Autodesk Inventor part; units mm, degrees
(part 4 of 4)
  line L444 (34, -62) -> (25.5, -62) projected
  line L445 (25.5, -62) -> (25.5, -60.5) projected
  line L446 (25.5, -60.5) -> (34, -60.5) projected
  line L447 (34, -60.5) -> (34, -62) projected
  line L448 (49, -32) -> (40.5, -32) projected
  line L449 (40.5, -32) -> (40.5, -30.5) projected
  line L450 (40.5, -30.5) -> (49, -30.5) projected
  line L451 (49, -30.5) -> (49, -32) projected
  line L452 (49, -62) -> (40.5, -62) projected
  line L453 (40.5, -62) -> (40.5, -60.5) projected
  line L454 (40.5, -60.5) -> (49, -60.5) projected
  line L455 (49, -60.5) -> (49, -62) projected
  line L456 (34, 60.5) -> (25.5, 60.5) projected
  line L457 (25.5, 60.5) -> (25.5, 62) projected
  line L458 (25.5, 62) -> (34, 62) projected
  line L459 (34, 62) -> (34, 60.5) projected
  line L460 (49, 58) -> (40.5, 58) projected
  line L461 (40.5, 58) -> (40.5, 59.5) projected
  line L462 (40.5, 59.5) -> (49, 59.5) projected
  line L463 (49, 59.5) -> (49, 58) projected
  line L464 (49, 45.5) -> (40.5, 45.5) projected
  line L465 (40.5, 45.5) -> (40.5, 47) projected
  line L466 (40.5, 47) -> (49, 47) projected
  line L467 (49, 47) -> (49, 45.5) projected
  line L468 (34, 30.5) -> (25.5, 30.5) projected
  line L469 (25.5, 30.5) -> (25.5, 32) projected
  line L470 (25.5, 32) -> (34, 32) projected
  line L471 (34, 32) -> (34, 30.5) projected
  line L472 (49, 43) -> (40.5, 43) projected
  line L473 (40.5, 43) -> (40.5, 44.5) projected
  line L474 (40.5, 44.5) -> (49, 44.5) projected
  line L475 (49, 44.5) -> (49, 43) projected
  line L476 (49, -2) -> (40.5, -2) projected
  line L477 (40.5, -2) -> (40.5, -0.5) projected
  line L478 (40.5, -0.5) -> (49, -0.5) projected
  line L479 (49, -0.5) -> (49, -2) projected
  line L480 (19, 103) -> (10.5, 103) projected
  line L481 (10.5, 103) -> (10.5, 104.5) projected
  line L482 (10.5, 104.5) -> (19, 104.5) projected
  line L483 (19, 104.5) -> (19, 103) projected
  line L484 (34, 103) -> (25.5, 103) projected
  line L485 (25.5, 103) -> (25.5, 104.5) projected
  line L486 (25.5, 104.5) -> (34, 104.5) projected
  line L487 (34, 104.5) -> (34, 103) projected
  line L488 (49, 103) -> (40.5, 103) projected
  line L489 (40.5, 103) -> (40.5, 104.5) projected
  line L490 (40.5, 104.5) -> (49, 104.5) projected
  line L491 (49, 104.5) -> (49, 103) projected
  line L492 (4, 103) -> (-4.5, 103) projected
  line L493 (-4.5, 103) -> (-4.5, 104.5) projected
  line L494 (-4.5, 104.5) -> (4, 104.5) projected
  line L495 (4, 104.5) -> (4, 103) projected
  line L496 (-11, 103) -> (-19.5, 103) projected
  line L497 (-19.5, 103) -> (-19.5, 104.5) projected
  line L498 (-19.5, 104.5) -> (-11, 104.5) projected
  line L499 (-11, 104.5) -> (-11, 103) projected
  line L500 (-26, 103) -> (-34.5, 103) projected
  line L501 (-34.5, 103) -> (-34.5, 104.5) projected
  line L502 (-34.5, 104.5) -> (-26, 104.5) projected
  line L503 (-26, 104.5) -> (-26, 103) projected
  line L504 (-41, 105.5) -> (-49.5, 105.5) projected
  line L505 (-49.5, 105.5) -> (-49.5, 107) projected
  line L506 (-49.5, 107) -> (-41, 107) projected
  line L507 (-41, 107) -> (-41, 105.5) projected
  line L508 (19, -84.5) -> (10.5, -84.5) projected
  line L509 (10.5, -84.5) -> (10.5, -83) projected
  line L510 (10.5, -83) -> (19, -83) projected
  line L511 (19, -83) -> (19, -84.5) projected
  line L512 (19, -39.5) -> (10.5, -39.5) projected
  line L513 (10.5, -39.5) -> (10.5, -38) projected
  line L514 (10.5, -38) -> (19, -38) projected
  line L515 (19, -38) -> (19, -39.5) projected
  line L516 (19, 20.5) -> (10.5, 20.5) projected
  line L517 (10.5, 20.5) -> (10.5, 22) projected
  line L518 (10.5, 22) -> (19, 22) projected
  line L519 (19, 22) -> (19, 20.5) projected
  line L520 (19, 65.5) -> (10.5, 65.5) projected
  line L521 (10.5, 65.5) -> (10.5, 67) projected
  line L522 (10.5, 67) -> (19, 67) projected
  line L523 (19, 67) -> (19, 65.5) projected
  line L524 (19, 43) -> (10.5, 43) projected
  line L525 (10.5, 43) -> (10.5, 44.5) projected
  line L526 (10.5, 44.5) -> (19, 44.5) projected
  line L527 (19, 44.5) -> (19, 43) projected
  line L528 (19, 5.5) -> (10.5, 5.5) projected
  line L529 (10.5, 5.5) -> (10.5, 7) projected
  line L530 (10.5, 7) -> (19, 7) projected
  line L531 (19, 7) -> (19, 5.5) projected
  line L532 (19, -62) -> (10.5, -62) projected
  line L533 (10.5, -62) -> (10.5, -60.5) projected
  line L534 (10.5, -60.5) -> (19, -60.5) projected
  line L535 (19, -60.5) -> (19, -62) projected
  line L536 (19, -99.5) -> (10.5, -99.5) projected
  line L537 (10.5, -99.5) -> (10.5, -98) projected
  line L538 (10.5, -98) -> (19, -98) projected
  line L539 (19, -98) -> (19, -99.5) projected
  line L540 (-26, 118) -> (-34.5, 118) projected
  line L541 (-34.5, 118) -> (-34.5, 119.5) projected
  line L542 (-34.5, 119.5) -> (-26, 119.5) projected
  line L543 (-26, 119.5) -> (-26, 118) projected
  line L544 (-11, 118) -> (-19.5, 118) projected
  line L545 (-19.5, 118) -> (-19.5, 119.5) projected
  line L546 (-19.5, 119.5) -> (-11, 119.5) projected
  line L547 (-11, 119.5) -> (-11, 118) projected
  line L548 (4, 118) -> (-4.5, 118) projected
  line L549 (-4.5, 118) -> (-4.5, 119.5) projected
  line L550 (-4.5, 119.5) -> (4, 119.5) projected
  line L551 (4, 119.5) -> (4, 118) projected
  line L552 (-41, 90.5) -> (-49.5, 90.5) projected
  line L553 (-49.5, 90.5) -> (-49.5, 92) projected
  line L554 (-49.5, 92) -> (-41, 92) projected
  line L555 (-41, 92) -> (-41, 90.5) projected
  line L556 (49, 118) -> (40.5, 118) projected
  line L557 (40.5, 118) -> (40.5, 119.5) projected
  line L558 (40.5, 119.5) -> (49, 119.5) projected
  line L559 (49, 119.5) -> (49, 118) projected
  line L560 (34, 118) -> (25.5, 118) projected
  line L561 (25.5, 118) -> (25.5, 119.5) projected
  line L562 (25.5, 119.5) -> (34, 119.5) projected
  line L563 (34, 119.5) -> (34, 118) projected
  line L564 (19, 118) -> (10.5, 118) projected
  line L565 (10.5, 118) -> (10.5, 119.5) projected
  line L566 (10.5, 119.5) -> (19, 119.5) projected
  line L567 (19, 119.5) -> (19, 118) projected
  line L568 (49, 28) -> (40.5, 28) projected
  line L569 (40.5, 28) -> (40.5, 29.5) projected
  line L570 (40.5, 29.5) -> (49, 29.5) projected
  line L571 (49, 29.5) -> (49, 28) projected
  line L572 (34, 15.5) -> (25.5, 15.5) projected
  line L573 (25.5, 15.5) -> (25.5, 17) projected
  line L574 (25.5, 17) -> (34, 17) projected
  line L575 (34, 17) -> (34, 15.5) projected
  line L576 (34, 45.5) -> (25.5, 45.5) projected
  line L577 (25.5, 45.5) -> (25.5, 47) projected
  line L578 (25.5, 47) -> (34, 47) projected
  line L579 (34, 47) -> (34, 45.5) projected
  line L580 (49, 0.5) -> (40.5, 0.5) projected
  line L581 (40.5, 0.5) -> (40.5, 2) projected
  line L582 (40.5, 2) -> (49, 2) projected
  line L583 (49, 2) -> (49, 0.5) projected
  line L584 (49, 73) -> (40.5, 73) projected
  line L585 (40.5, 73) -> (40.5, 74.5) projected
  line L586 (40.5, 74.5) -> (49, 74.5) projected
  line L587 (49, 74.5) -> (49, 73) projected
  line L588 (34, 75.5) -> (25.5, 75.5) projected
  line L589 (25.5, 75.5) -> (25.5, 77) projected
  line L590 (25.5, 77) -> (34, 77) projected
  line L591 (34, 77) -> (34, 75.5) projected
  line L592 (49, -47) -> (40.5, -47) projected
  line L593 (40.5, -47) -> (40.5, -45.5) projected
  line L594 (40.5, -45.5) -> (49, -45.5) projected
  line L595 (49, -45.5) -> (49, -47) projected
  line L596 (49, -17) -> (40.5, -17) projected
  line L597 (40.5, -17) -> (40.5, -15.5) projected
  line L598 (40.5, -15.5) -> (49, -15.5) projected
  line L599 (49, -15.5) -> (49, -17) projected
  line L600 (34, -47) -> (25.5, -47) projected
  line L601 (25.5, -47) -> (25.5, -45.5) projected
  line L602 (25.5, -45.5) -> (34, -45.5) projected
  line L603 (34, -45.5) -> (34, -47) projected
  line L604 (34, -14.5) -> (25.5, -14.5) projected
  line L605 (25.5, -14.5) -> (25.5, -13) projected
  line L606 (25.5, -13) -> (34, -13) projected
  line L607 (34, -13) -> (34, -14.5) projected
  line L608 (49, -104.5) -> (40.5, -104.5) projected
  line L609 (40.5, -104.5) -> (40.5, -103) projected
  line L610 (40.5, -103) -> (49, -103) projected
  line L611 (49, -103) -> (49, -104.5) projected
  line L612 (34, -119.5) -> (25.5, -119.5) projected
  line L613 (25.5, -119.5) -> (25.5, -118) projected
  line L614 (25.5, -118) -> (34, -118) projected
  line L615 (34, -118) -> (34, -119.5) projected
  line L616 (34, -74.5) -> (25.5, -74.5) projected
  line L617 (25.5, -74.5) -> (25.5, -73) projected
  line L618 (25.5, -73) -> (34, -73) projected
  line L619 (34, -73) -> (34, -74.5) projected
  line L620 (34, 88) -> (25.5, 88) projected
  line L621 (25.5, 88) -> (25.5, 89.5) projected
  line L622 (25.5, 89.5) -> (34, 89.5) projected
  line L623 (34, 89.5) -> (34, 88) projected
  line L624 (-11, -17) -> (-19.5, -17) projected
  line L625 (-19.5, -17) -> (-19.5, -15.5) projected
  line L626 (-19.5, -15.5) -> (-11, -15.5) projected
  line L627 (-11, -15.5) -> (-11, -17) projected
  line L628 (-11, -59.5) -> (-19.5, -59.5) projected
  line L629 (-19.5, -59.5) -> (-19.5, -58) projected
  line L630 (-19.5, -58) -> (-11, -58) projected
  line L631 (-11, -58) -> (-11, -59.5) projected
  line L632 (4, -62) -> (-4.5, -62) projected
  line L633 (-4.5, -62) -> (-4.5, -60.5) projected
  line L634 (-4.5, -60.5) -> (4, -60.5) projected
  line L635 (4, -60.5) -> (4, -62) projected
  line L636 (-11, -44.5) -> (-19.5, -44.5) projected
  line L637 (-19.5, -44.5) -> (-19.5, -43) projected
  line L638 (-19.5, -43) -> (-11, -43) projected
  line L639 (-11, -43) -> (-11, -44.5) projected
  line L640 (-11, -77) -> (-19.5, -77) projected
  line L641 (-19.5, -77) -> (-19.5, -75.5) projected
  line L642 (-19.5, -75.5) -> (-11, -75.5) projected
  line L643 (-11, -75.5) -> (-11, -77) projected
  line L644 (-11, -107) -> (-19.5, -107) projected
  line L645 (-19.5, -107) -> (-19.5, -105.5) projected
  line L646 (-19.5, -105.5) -> (-11, -105.5) projected
  line L647 (-11, -105.5) -> (-11, -107) projected
  line L648 (4, -89.5) -> (-4.5, -89.5) projected
  line L649 (-4.5, -89.5) -> (-4.5, -88) projected
  line L650 (-4.5, -88) -> (4, -88) projected
  line L651 (4, -88) -> (4, -89.5) projected
  line L652 (4, -104.5) -> (-4.5, -104.5) projected
  line L653 (-4.5, -104.5) -> (-4.5, -103) projected
  line L654 (-4.5, -103) -> (4, -103) projected
  line L655 (4, -103) -> (4, -104.5) projected
  line L656 (19, -119.5) -> (10.5, -119.5) projected
  line L657 (10.5, -119.5) -> (10.5, -118) projected
  line L658 (10.5, -118) -> (19, -118) projected
  line L659 (19, -118) -> (19, -119.5) projected
  line L660 (19, 88) -> (10.5, 88) projected
  line L661 (10.5, 88) -> (10.5, 89.5) projected
  line L662 (10.5, 89.5) -> (19, 89.5) projected
  line L663 (19, 89.5) -> (19, 88) projected
  line L664 (4, -77) -> (-4.5, -77) projected
  line L665 (-4.5, -77) -> (-4.5, -75.5) projected
  line L666 (-4.5, -75.5) -> (4, -75.5) projected
  line L667 (4, -75.5) -> (4, -77) projected
  line L668 (-11, -119.5) -> (-19.5, -119.5) projected
  line L669 (-19.5, -119.5) -> (-19.5, -118) projected
  line L670 (-19.5, -118) -> (-11, -118) projected
  line L671 (-11, -118) -> (-11, -119.5) projected
  line L672 (-11, -89.5) -> (-19.5, -89.5) projected
  line L673 (-19.5, -89.5) -> (-19.5, -88) projected
  line L674 (-19.5, -88) -> (-11, -88) projected
  line L675 (-11, -88) -> (-11, -89.5) projected
  line L676 (4, -59.5) -> (-4.5, -59.5) projected
  line L677 (-4.5, -59.5) -> (-4.5, -58) projected
  line L678 (-4.5, -58) -> (4, -58) projected
  line L679 (4, -58) -> (4, -59.5) projected
  line L680 (4, -29.5) -> (-4.5, -29.5) projected
  line L681 (-4.5, -29.5) -> (-4.5, -28) projected
  line L682 (-4.5, -28) -> (4, -28) projected
  line L683 (4, -28) -> (4, -29.5) projected
  line L684 (-11, -62) -> (-19.5, -62) projected
  line L685 (-19.5, -62) -> (-19.5, -60.5) projected
  line L686 (-19.5, -60.5) -> (-11, -60.5) projected
  line L687 (-11, -60.5) -> (-11, -62) projected
  line L688 (-11, -29.5) -> (-19.5, -29.5) projected
  line L689 (-19.5, -29.5) -> (-19.5, -28) projected
  line L690 (-19.5, -28) -> (-11, -28) projected
  line L691 (-11, -28) -> (-11, -29.5) projected
  line L692 (-11, -2) -> (-19.5, -2) projected
  line L693 (-19.5, -2) -> (-19.5, -0.5) projected
  line L694 (-19.5, -0.5) -> (-11, -0.5) projected
  line L695 (-11, -0.5) -> (-11, -2) projected
  line L696 (34, -104.5) -> (25.5, -104.5) projected
  line L697 (25.5, -104.5) -> (25.5, -103) projected
  line L698 (25.5, -103) -> (34, -103) projected
  line L699 (34, -103) -> (34, -104.5) projected
  line L700 (34, -92) -> (25.5, -92) projected
  line L701 (25.5, -92) -> (25.5, -90.5) projected
  line L702 (25.5, -90.5) -> (34, -90.5) projected
  line L703 (34, -90.5) -> (34, -92) projected
  line L704 (49, -89.5) -> (40.5, -89.5) projected
  line L705 (40.5, -89.5) -> (40.5, -88) projected
  line L706 (40.5, -88) -> (49, -88) projected
  line L707 (49, -88) -> (49, -89.5) projected
  line L708 (34, -29.5) -> (25.5, -29.5) projected
  line L709 (25.5, -29.5) -> (25.5, -28) projected
  line L710 (25.5, -28) -> (34, -28) projected
  line L711 (34, -28) -> (34, -29.5) projected
  line L712 (34, -44.5) -> (25.5, -44.5) projected
  line L713 (25.5, -44.5) -> (25.5, -43) projected
  line L714 (25.5, -43) -> (34, -43) projected
  line L715 (34, -43) -> (34, -44.5) projected
  line L716 (49, -14.5) -> (40.5, -14.5) projected
  line L717 (40.5, -14.5) -> (40.5, -13) projected
  line L718 (40.5, -13) -> (49, -13) projected
  line L719 (49, -13) -> (49, -14.5) projected
  line L720 (49, -44.5) -> (40.5, -44.5) projected
  line L721 (40.5, -44.5) -> (40.5, -43) projected
  line L722 (40.5, -43) -> (49, -43) projected
  line L723 (49, -43) -> (49, -44.5) projected
  line L724 (34, 58) -> (25.5, 58) projected
  line L725 (25.5, 58) -> (25.5, 59.5) projected
  line L726 (25.5, 59.5) -> (34, 59.5) projected
  line L727 (34, 59.5) -> (34, 58) projected
  line L728 (49, 75.5) -> (40.5, 75.5) projected
  line L729 (40.5, 75.5) -> (40.5, 77) projected
  line L730 (40.5, 77) -> (49, 77) projected
  line L731 (49, 77) -> (49, 75.5) projected
  line L732 (49, 13) -> (40.5, 13) projected
  line L733 (40.5, 13) -> (40.5, 14.5) projected
  line L734 (40.5, 14.5) -> (49, 14.5) projected
  line L735 (49, 14.5) -> (49, 13) projected
  line L736 (34, -2) -> (25.5, -2) projected
  line L737 (25.5, -2) -> (25.5, -0.5) projected
  line L738 (25.5, -0.5) -> (34, -0.5) projected
  line L739 (34, -0.5) -> (34, -2) projected
  line L740 (34, 28) -> (25.5, 28) projected
  line L741 (25.5, 28) -> (25.5, 29.5) projected
  line L742 (25.5, 29.5) -> (34, 29.5) projected
  line L743 (34, 29.5) -> (34, 28) projected
  line L744 (49, 30.5) -> (40.5, 30.5) projected
  line L745 (40.5, 30.5) -> (40.5, 32) projected
  line L746 (40.5, 32) -> (49, 32) projected
  line L747 (49, 32) -> (49, 30.5) projected
  line L748 (49, 88) -> (40.5, 88) projected
  line L749 (40.5, 88) -> (40.5, 89.5) projected
  line L750 (40.5, 89.5) -> (49, 89.5) projected
  line L751 (49, 89.5) -> (49, 88) projected
  line L752 (19, 90.5) -> (10.5, 90.5) projected
  line L753 (10.5, 90.5) -> (10.5, 92) projected
  line L754 (10.5, 92) -> (19, 92) projected
  line L755 (19, 92) -> (19, 90.5) projected
  line L756 (34, 90.5) -> (25.5, 90.5) projected
  line L757 (25.5, 90.5) -> (25.5, 92) projected
  line L758 (25.5, 92) -> (34, 92) projected
  line L759 (34, 92) -> (34, 90.5) projected
  line L760 (49, 90.5) -> (40.5, 90.5) projected
  line L761 (40.5, 90.5) -> (40.5, 92) projected
  line L762 (40.5, 92) -> (49, 92) projected
  line L763 (49, 92) -> (49, 90.5) projected
  line L764 (4, 105.5) -> (-4.5, 105.5) projected
  line L765 (-4.5, 105.5) -> (-4.5, 107) projected
  line L766 (-4.5, 107) -> (4, 107) projected
  line L767 (4, 107) -> (4, 105.5) projected
  line L768 (-11, 105.5) -> (-19.5, 105.5) projected
  line L769 (-19.5, 105.5) -> (-19.5, 107) projected
  line L770 (-19.5, 107) -> (-11, 107) projected
  line L771 (-11, 107) -> (-11, 105.5) projected
  line L772 (-26, 105.5) -> (-34.5, 105.5) projected
  line L773 (-34.5, 105.5) -> (-34.5, 107) projected
  line L774 (-34.5, 107) -> (-26, 107) projected
  line L775 (-26, 107) -> (-26, 105.5) projected
  line L776 (-41, 118) -> (-49.5, 118) projected
  line L777 (-49.5, 118) -> (-49.5, 119.5) projected
  line L778 (-49.5, 119.5) -> (-41, 119.5) projected
  line L779 (-41, 119.5) -> (-41, 118) projected
  line L780 (19, -82) -> (10.5, -82) projected
  line L781 (10.5, -82) -> (10.5, -80.5) projected
  line L782 (10.5, -80.5) -> (19, -80.5) projected
  line L783 (19, -80.5) -> (19, -82) projected
  line L784 (19, -37) -> (10.5, -37) projected
  line L785 (10.5, -37) -> (10.5, -35.5) projected
  line L786 (10.5, -35.5) -> (19, -35.5) projected
  line L787 (19, -35.5) -> (19, -37) projected
  line L788 (19, 23) -> (10.5, 23) projected
  line L789 (10.5, 23) -> (10.5, 24.5) projected
  line L790 (10.5, 24.5) -> (19, 24.5) projected
  line L791 (19, 24.5) -> (19, 23) projected
  line L792 (19, 68) -> (10.5, 68) projected
  line L793 (10.5, 68) -> (10.5, 69.5) projected
  line L794 (10.5, 69.5) -> (19, 69.5) projected
  line L795 (19, 69.5) -> (19, 68) projected
  circle A15 centre (-56, 65.75) radius 1.75 projected
  circle A16 centre (56, -65.75) radius 1.75 projected
  circle A17 centre (56, 65.75) radius 1.75 projected
  circle A18 centre (-56, -65.75) radius 1.75 projected
  line L796 (4.75, 10) -> (4.75, 43.5) projected
  line L797 (4.75, 43.5) -> (-0.25, 43.5) projected
  line L798 (-0.25, 43.5) -> (-0.25, 10) projected
  line L799 (-0.25, 10) -> (4.75, 10) projected
  line L800 (5.5, 63) -> (5.5, 5.75) projected
  line L801 (4.5, 5.75) -> (4.5, 9.75) projected
  line L802 (5.5, 5.75) -> (4.5, 5.75)
  line L803 (4.5, 5.75) -> (4.5, 9.75)
  line L804 (4.5, 9.75) -> (5.5, 9.75)
  line L805 (5.5, 9.75) -> (5.5, 5.75)
  line L806 (5.5, 63) -> (-34.5, 63) projected
  line L807 (-52.25, 1.75) -> (-52.25, 88.25) projected
  line L808 (-1.25, 63) -> (-52.25, 63)
  line L809 (-52.25, 63) -> (-52.25, 9.75)
  line L810 (-52.25, 9.75) -> (-1.25, 9.75)
  line L811 (-1.25, 9.75) -> (-1.25, 63)
  line L812 (-44.5, 1.75) -> (-52.25, 1.75) projected
  line L813 (-44.5, 1.75) -> (-52.25, 1.75)
  line L814 (-52.25, 1.75) -> (-52.25, 9.75)
  line L815 (-52.25, 9.75) -> (-44.5, 9.75)
  line L816 (-44.5, 9.75) -> (-44.5, 1.75)
  line L817 (-52.25, 88.25) -> (-34.5, 88.25) projected
  line L818 (-34.5, 63) -> (-52.25, 63)
  line L819 (-52.25, 63) -> (-52.25, 88.25)
  line L820 (-52.25, 88.25) -> (-34.5, 88.25)
  line L821 (-34.5, 88.25) -> (-34.5, 63)
  line L822 (-52.25, 68.25) -> (-37.25, 68.25)
  line L823 (-37.25, 68.25) -> (-37.25, 21.75)
  line L824 (-37.25, 21.75) -> (-52.25, 21.75)
  line L825 (-52.25, 21.75) -> (-52.25, 68.25)
  point P0 (0, 0)
  point P1 (-1.25, 9.75)
  dimension "d510" = 1
  dimension "d511" = 20
  dimension "d512" = 20
  dimension "d513" = 15
  constraints: 40 end point, 10 parallel, 5 horizontal, 5 perpendicular, 4 point on line
  measures "d510" distance between parallel lines of L811 L798
  measures "d511" distance between parallel lines of L817 L822
  measures "d512" distance between parallel lines of L0 L824
  measures "d513" distance between parallel lines of L1 L823
extrude "Extrusion21" add sketch "Sketch42" against normal up to surface (4 mm away) contours L0 L1 L810 L9 | L810 L1 L824 L823 L808 L4 L811 L8 | L804 L5 L6 L7 | L808 L823 L822 L1 L2 L3
body "Solid1"
